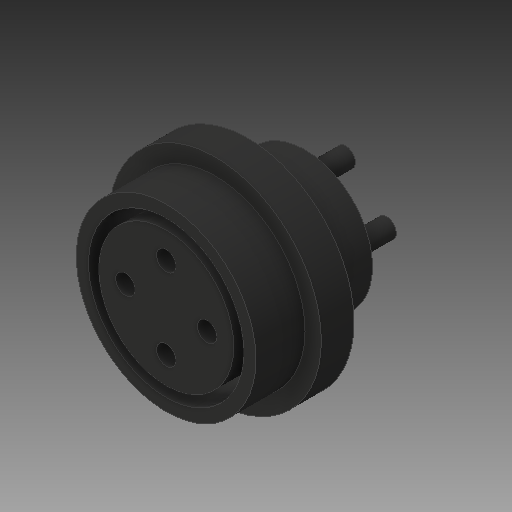
# Autodesk Inventor part: connector
Saved by Autodesk Inventor 2018.1 (Build 221171000, 171)
## iProperties
Created: 2017-08-10
Part Number: connector
Material: Rubber
Document SubType Name: Modeling
Designer: Kai
Density: 0.93 g/cm^3
Appearance: Rubber - Black
Author: Kai
Autodesk Inventor part; units mm, degrees
ref_plane "YZ Plane" through (0, 0, 0) normal (1, 0, 0) x (0, 1, 0)
ref_plane "XZ Plane" through (0, 0, 0) normal (0, 1, 0) x (-1, 0, 0)
ref_plane "XY Plane" through (0, 0, 0) normal (0, 0, 1) x (1, 0, 0)
sketch "Sketch1" plane through (0, 0, 0) normal (0, 0, 1) x (1, 0, 0)
  circle A0 centre (0, 0) radius 10.5
  dimension "d0" = 21
  constraints: 1 centre point, 1 coincident
  measures "d0" diameter of A0
extrude "Extrusion1" add sketch "Sketch1" along normal blind 8.89
sketch "Sketch2" plane through (0, 0, 8.89) normal (0, 0, 1) x (1, 0, 0)
  circle A0 centre (0, 0) radius 16.51
  dimension "d3" = 33.02
  constraints: 1 centre point, 1 coincident
  measures "d3" diameter of A0
extrude "Extrusion2" add sketch "Sketch2" along normal blind 5.08
sketch "Sketch3" plane through (0, 0, 13.97) normal (0, 0, 1) x (1, 0, 0)
  circle A0 centre (0, 0) radius 13.97
  dimension "d6" = 27.94
  constraints: 1 centre point, 1 coincident
  measures "d6" diameter of A0
extrude "Extrusion3" add sketch "Sketch3" along normal blind 7.62
sketch "Sketch4" plane through (0, 0, 21.59) normal (0, 0, 1) x (1, 0, 0)
  circle A0 centre (0, 0) radius 6.35 construction
  circle A1 centre (0, 6.35) radius 1.5
  circle A2 centre (-6.35, 0) radius 1.5
  circle A3 centre (0, -6.35) radius 1.5
  circle A4 centre (6.35, 0) radius 1.5
  dimension "d9" = 12.7
  dimension "d10" = 3
  dimension "d13" = 360
  constraints: 4 centre point, 1 coincident, 1 vertical alignment, 11 other
  measures "d10" diameter of A1
extrude "Extrusion4" cut sketch "Sketch4" against normal blind 11.43
sketch "Sketch5" plane through (0, 0, 21.59) normal (0, 0, 1) x (1, 0, 0)
  circle A0 centre (0, 0) radius 10.5
  circle A1 centre (0, 0) radius 10.5 projected
  circle A2 centre (0, 0) radius 12.065
  dimension "d17" = 24.13
  constraints: 2 centre point, 2 coincident
  measures "d17" diameter of A2
extrude "Extrusion5" cut sketch "Sketch5" against normal blind 11.43
sketch "Sketch6" plane through (0, 0, 0) normal (0, 0, -1) x (-1, 0, 0)
  circle A0 centre (0, 6.35) radius 1.5 projected
  circle A1 centre (0, 0) radius 6.35 construction
  circle A2 centre (0, 6.35) radius 1.5
  circle A3 centre (0, 0) radius 6.35 construction
  circle A4 centre (-6.35, 0) radius 1.5
  circle A5 centre (0, 0) radius 6.35 construction
  circle A6 centre (0, -6.35) radius 1.5
  circle A7 centre (0, 0) radius 6.35 construction
  circle A8 centre (6.35, 0) radius 1.5
  dimension "d22" = 360
  constraints: 5 coincident, 4 centre point, 2 horizontal alignment, 2 vertical alignment, 1 concentric, 29 other
extrude "Extrusion6" add sketch "Sketch6" along normal blind 6.35
body "Solid1"
